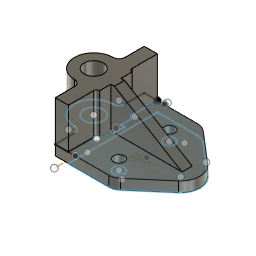
A2 v1 (Autodesk Fusion 360 design; units mm, degrees)
Autodesk Fusion 360 part; units mm, degrees
sketch "Base 1" plane through (0, 0, 0) normal (0, 0, 1) x (1, 0, 0)
  line L0 (6.4814, 44) -> (-33.5, 44)
  line L1 (-33.5, 44) -> (-33.5, -44)
  line L2 (-33.5, -44) -> (6.4814, -44)
  line L3 (-33.5, -25) -> (-33.5, 25) construction
  line L4 (45.8485, -14.44) -> (14.9304, -40.88)
  line L5 (33.5, 25) -> (45.8485, 14.44) construction
  line L6 (14.9304, 40.88) -> (45.8485, 14.44)
  arc A0 (6.4814, -44) -> (14.9304, -40.88) centre (6.4814, -31) ccw
  arc A1 (14.9304, 40.88) -> (6.4814, 44) centre (6.4814, 31) ccw
  circle A2 centre (-2.5, -25) radius 5.3151
  circle A3 centre (-2.5, 25) radius 5.3151
  arc A4 (45.8485, -14.44) -> (45.8485, 14.44) centre (33.5, 0) ccw
  dimension "d2" = 88
  dimension "d4" = 50
  dimension "d6" = 38
  dimension "d7" = 13
  dimension "d8" = 13
  dimension "d9" = 31
  dimension "d10" = 10.6301
  constraint horizontal L0
  constraint perpendicular L0 L1
  constraint parallel L0 L2
  constraint vertical L3
  constraint coincident L1 L3.end
  constraint tangent L5 A4
  constraint tangent L2 A0
  constraint tangent L4 A0
  constraint tangent L0 A1
  constraint tangent L6 A1
  measures "d2" distance of L0.end L1.end
  measures "d4" distance of L3.end L3.start
  measures "d6" diameter of A4
  measures "d7" radius of A0
  measures "d8" radius of A1
  measures "d9" distance of L3.start A2.centre
  measures "d10" diameter of A2
extrude "Extrude1" add sketch "Base 1" along normal blind 10
sketch "Base 2" plane through (0, 0, 10) normal (0, 0, 1) x (-1, 0, 0)
  circle A0 centre (2.5, 25) radius 5.3151
  circle A1 centre (2.5, -25) radius 5.3151
  arc A2 (-14.9304, -40.88) -> (-6.4814, -44) centre (-6.4814, -31) ccw
  line L0 (-6.4814, -44) -> (33.5, -44)
  line L1 (33.5, -44) -> (33.5, 44)
  line L2 (33.5, 44) -> (-6.4814, 44)
  arc A3 (-6.4814, 44) -> (-14.9304, 40.88) centre (-6.4814, 31) ccw
  line L3 (-14.9304, 40.88) -> (-45.8485, 14.44)
  arc A4 (-45.8485, 14.44) -> (-45.8485, -14.44) centre (-33.5, 0) ccw
  line L4 (-45.8485, -14.44) -> (-14.9304, -40.88)
  line L5 (33.5, -44) -> (46.5, -44)
  line L6 (46.5, -44) -> (46.5, -25)
  line L7 (46.5, 44) -> (33.5, 44)
  line L8 (33.5, 44) -> (33.5, 19)
  line L9 (30.5, 16) -> (30.5, 16)
  line L10 (30.5, -16) -> (30.5, -16)
  arc A5 (30.5, 16) -> (33.5, 19) centre (30.5, 19) ccw
  line L11 (33.5, -44) -> (33.5, -19)
  arc A6 (33.5, -19) -> (30.5, -16) centre (30.5, -19) ccw
  circle A7 centre (52.5, 0) radius 9.5
  line L12 (52.5, -19) -> (52.5, -19) construction
  arc A8 (52.5, -19) -> (46.5, -25) centre (52.5, -25) ccw
  line L13 (46.5, 25) -> (46.5, 44)
  line L14 (52.5, 19) -> (52.5, 19) construction
  arc A9 (46.5, 25) -> (52.5, 19) centre (52.5, 25) ccw
  line L15 (27, -5) -> (30.5, -5) construction
  line L16 (27, 5) -> (27, -5) construction
  line L17 (30.5, -5) -> (27, -5)
  line L18 (27, -5) -> (27, 5)
  line L19 (27, 5) -> (30.5, 5)
  line L20 (30.5, -16) -> (30.5, -5)
  line L21 (30.5, 5) -> (30.5, 16)
  arc A10 (52.5, -19) -> (52.5, 19) centre (52.5, 0) ccw
  line L22 (26.5, -46.8903) -> (26.5, -44) construction
  line L23 (26.5, 44) -> (26.5, 65) construction
  line L24 (30.5, 5) -> (27, 5) construction
  point P0 (30.5, 0)
  dimension "d13" = 13
  dimension "d14" = 88
  dimension "d17" = 3
  dimension "d18" = 3
  dimension "d20" = 19
  dimension "d21" = 38
  dimension "d22" = 6
  dimension "d23" = 6
  constraint horizontal L5
  constraint vertical L6
  constraint horizontal L7
  constraint vertical L8
  constraint coincident L0.end L1.start
  constraint coincident L0.end L8
  constraint tangent L8 A5
  constraint tangent L11 A6
  constraint concentric A7 A10
  constraint coincident L7.start L6
  constraint tangent L6 A8
  constraint coincident L6.end L13
  constraint tangent L13 A9
  constraint perpendicular L2 L22
  constraint horizontal L15
  constraint perpendicular L19 L20
  constraint collinear L20 L21
  constraint coincident P0 L20
  constraint coincident L0 L22.end
  constraint coincident L2 L23.start
  constraint collinear L22 L23
  measures "d13" distance of L0.end L5.end
  measures "d14" distance of L0.end L1.end
  measures "d17" radius of A5
  measures "d18" radius of A6
  measures "d20" diameter of A7
  measures "d21" diameter of A10
  measures "d22" radius of A8
  measures "d23" radius of A9
extrude "Extrude2" add sketch "Base 2" against normal blind 10 contours L1 L5 L6 L7 L8 L11 A8 L13 A9 A10
extrude "Extrude3" add sketch "Base 2" along normal blind 40 contours L1 L5 L6 L7 L8 L11 A8 L13 A9 A10
extrude "Extrude4" add sketch "Base 2" along normal blind 40 contours L1 A5 A6 L17 L18 L19 L20 L21
sketch "Triangle" plane through (0, 0, 0) normal (0, 1, 0) x (1, 0, 0)
  line L0 (-27, -10) -> (40, -10)
  line L1 (40, -10) -> (-27, -50)
  line L2 (-27, -50) -> (-27, -10)
  dimension "d32" = 67
  constraint horizontal L0
  constraint perpendicular L0 L2
  measures "d32" distance of L0.start L0.end
extrude "Extrude5" add sketch "Triangle" along normal mid plane 10
